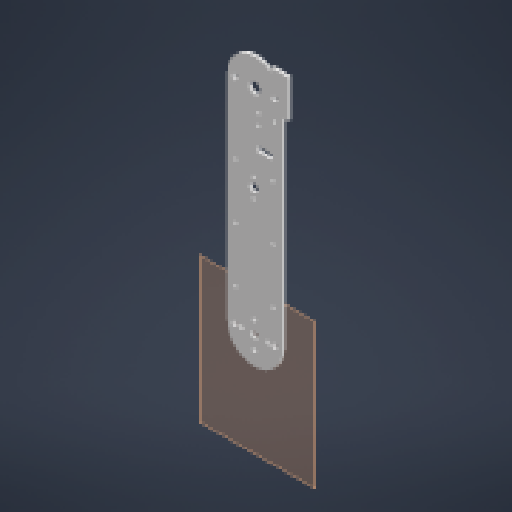
# Autodesk Inventor part: Link2Base
Saved by Autodesk Inventor 2023 (Build 270158000, 158)
## iProperties
Created: 2023-09-09
Part Number: Link2Base
Material: Generic
Document SubType Name: Modeling
Designer: philo
Density: 1 g/cm^3
Appearance: Default
Author: philo
Autodesk Inventor part; units mm, degrees
ref_plane "YZ Plane" through (0, 0, 0) normal (1, 0, 0) x (0, 1, 0)
ref_plane "XZ Plane" through (0, 0, 0) normal (0, 1, 0) x (-1, 0, 0)
ref_plane "XY Plane" through (0, 0, 0) normal (0, 0, 1) x (1, 0, 0)
ref_plane "Work Plane2" through (0.4904, 0, 14) normal (0, 0, 1) x (1, 0, 0)
sketch "Sketch1" plane through (0.4904, 0, 14) normal (0, 0, 1) x (1, 0, 0)
  line L0 (-25, 225.7065) -> (25, 225.7065)
  line L1 (25, 225.7065) -> (25, 5.7065)
  line L2 (25, 5.7065) -> (-25, 5.7065)
  line L3 (-25, 5.7065) -> (-25, 225.7065)
  line L4 (-25, 225.7065) -> (25, 225.7065)
  line L5 (20, 5.7065) -> (-20, 5.7065)
  circle A0 centre (0, 30.7065) radius 3.5 projected
  circle A1 centre (0, 30.7065) radius 25
  circle A2 centre (0, 225.7065) radius 25
  line L6 (-25, 30.7065) -> (-25, 225.7065)
  line L7 (25, 225.7065) -> (25, 30.7065)
  point P0 (-0.4904, 0)
  dimension "d19" = 50
  dimension "d6" = 220
  dimension "d7" = 0
  dimension "d9" = 50
  dimension "d10" = 25
  dimension "d11" = 25
  dimension "d12" = 25
  dimension "d13" = 0
  constraints: 16 end point, 3 parallel, 2 horizontal, 2 point on circle, 2 point on line, 1 centre point, 1 coincident, 1 midpoint, 1 perpendicular, 3 other
  measures "d6" distance between parallel lines of L2 L0
  measures "d7" distance between parallel lines of L0 L4
  measures "d9" diameter of A1
  measures "d10" distance from line of L3 A1.centre
  measures "d11" distance from line of L1 A1.centre
  measures "d12" distance from line of A1.centre L2
  measures "d13" distance between parallel lines of L5 L2
extrude "Extrusion1" add sketch "Sketch1" along normal blind 3 contours A2 L0 | A2 L1 A1 L3 | L0 A2 | A1
sketch "Sketch2" plane through (0.4904, 0, 17) normal (0, 0, 1) x (1, 0, 0)
  arc A0 (25, 225.7065) -> (-25, 225.7065) centre (0, 225.7065) ccw projected
  circle A1 centre (0, 225.7065) radius 5
  point P0 (-0.4904, 0)
  dimension "d16" = 10
  constraints: 1 centre point, 1 coincident
  measures "d16" diameter of A1
extrude "Extrusion2" cut sketch "Sketch2" against normal blind 3
sketch "Sketch4" plane through (0.4904, 0, 17) normal (0, 0, 1) x (1, 0, 0)
  arc A0 (20.4946, 25.2317) -> (20.5054, 36.1404) centre (18, 30.6886) ccw projected
  line L0 (20.5054, 36.1404) -> (10.4453, 40.7636) projected
  arc A1 (10.4252, 20.6286) -> (10.4453, 40.7636) centre (0, 30.7065) ccw projected
  line L1 (10.4252, 20.6286) -> (20.4946, 25.2317) projected
  circle A2 centre (18, 30.6886) radius 2.5 projected
  arc A3 (-20.5376, 36.019) -> (-20.4622, 25.1105) centre (-18, 30.582) ccw projected
  line L2 (-20.4622, 25.1105) -> (-11.0226, 20.8627) projected
  arc A4 (-11.1577, 40.3969) -> (-11.0226, 20.8627) centre (0, 30.7065) ccw projected
  line L3 (-11.1577, 40.3969) -> (-20.5376, 36.019) projected
  circle A5 centre (-18, 30.582) radius 2.5 projected
  point P0 (-0.4904, 0)
extrude "Extrusion4" cut sketch "Sketch4" against normal blind 10 contours A2 | A5
sketch "Sketch6" plane through (0.4904, 0, 14) normal (0, 0, -1) x (-1, 0, 0)
  circle A0 centre (0, 42.7065) radius 2 projected
  circle A1 centre (-12, 30.7065) radius 2 projected
  circle A2 centre (0, 18.7065) radius 2 projected
  circle A3 centre (12, 30.7065) radius 2 projected
  point P0 (0.4904, 0)
extrude "Extrusion6" cut sketch "Sketch6" against normal blind 10
sketch "Sketch7" plane through (0.4904, 0, 14) normal (0, 0, -1) x (-1, 0, 0)
  circle A0 centre (-12, 30.7065) radius 2 projected
  circle A1 centre (0, 18.7065) radius 2 projected
  circle A2 centre (12, 30.7065) radius 2 projected
  circle A3 centre (0, 42.7065) radius 2 projected
  circle A4 centre (-18, 30.6886) radius 2.5 projected
  circle A5 centre (18, 30.582) radius 2.5 projected
  circle A6 centre (0, 225.7065) radius 5 projected
  line L0 (25, 225.7065) -> (25, 30.7065) projected
  line L1 (-25, 30.7065) -> (-25, 225.7065) projected
  arc A7 (-25, 30.7065) -> (25, 30.7065) centre (0, 30.7065) ccw projected
  circle A8 centre (0, 30.7065) radius 3.5 projected
  circle A9 centre (0.668, 146.5279) radius 12.5 projected
  circle A10 centre (9.168, 146.5279) radius 2.3813 projected
  circle A11 centre (-7.832, 146.5279) radius 2.3813 projected
  circle A12 centre (0.668, 155.0279) radius 1.5 projected
  circle A13 centre (0.668, 138.0279) radius 1.5 projected
  circle A14 centre (0.668, 146.5279) radius 4
  arc A15 (25, 225.7065) -> (-25, 225.7065) centre (0, 225.7065) ccw projected
  point P0 (0.4904, 0)
  dimension "d60" = 8
  constraints: 1 centre point, 1 coincident
  measures "d60" diameter of A14
extrude "Extrusion7" cut sketch "Sketch7" against normal blind 10 contours A12 | A13 | A14
sketch "Sketch10" plane through (0.4904, 0, 17) normal (0, 0, 1) x (1, 0, 0)
  line L0 (17, 181.6543) -> (2, 181.6543)
  line L1 (2, 181.6543) -> (2, 176.6543)
  line L2 (2, 176.6543) -> (17, 176.6543)
  line L3 (17, 176.6543) -> (17, 181.6543)
  line L4 (25, 30.7065) -> (25, 225.7065) projected
  point P0 (-0.4904, 0)
  dimension "d67" = 15
  dimension "d68" = 5
  dimension "d69" = 8
  constraints: 8 end point, 2 parallel, 1 horizontal, 1 perpendicular
  measures "d67" distance of L2.end L1.end
  measures "d68" distance of L1.end L0.end
  measures "d69" distance between parallel lines of L4 L3
extrude "Extrusion10" cut sketch "Sketch10" against normal blind 10
fillet "Fillet1" radius 2 4 edges at (17.4904, 176.6543, 15.5) (17.4904, 181.6543, 15.5) (2.4904, 181.6543, 15.5) (2.4904, 176.6543, 15.5)
sketch "Sketch11" plane through (0.4904, 0, 17) normal (0, 0, 1) x (1, 0, 0)
  arc A0 (20.5376, 220.3941) -> (20.4622, 231.3026) centre (18, 225.831) ccw projected
  line L0 (20.4622, 231.3026) -> (11.0226, 235.5503) projected
  arc A1 (11.1577, 216.0162) -> (11.0226, 235.5503) centre (0, 225.7065) ccw projected
  line L1 (11.1577, 216.0162) -> (20.5376, 220.3941) projected
  circle A2 centre (18, 225.831) radius 2.5 projected
  arc A3 (-20.4946, 231.1813) -> (-20.5054, 220.2726) centre (-18, 225.7245) ccw projected
  line L2 (-20.5054, 220.2726) -> (-10.4453, 215.6494) projected
  arc A4 (-10.4252, 235.7844) -> (-10.4453, 215.6494) centre (0, 225.7065) ccw projected
  line L3 (-10.4252, 235.7844) -> (-20.4946, 231.1813) projected
  circle A5 centre (-18, 225.7245) radius 2.5 projected
  circle A6 centre (3.5, 208.0565) radius 1.5 projected
  circle A7 centre (3.5, 197.2565) radius 1.5 projected
  line L4 (15, 176.6543) -> (4, 176.6543) projected
  arc A8 (2, 178.6543) -> (4, 176.6543) centre (4, 178.6543) ccw projected
  line L5 (2, 178.6543) -> (2, 179.6543) projected
  arc A9 (4, 181.6543) -> (2, 179.6543) centre (4, 179.6543) ccw projected
  line L6 (4, 181.6543) -> (15, 181.6543) projected
  arc A10 (17, 179.6543) -> (15, 181.6543) centre (15, 179.6543) ccw projected
  line L7 (17, 179.6543) -> (17, 178.6543) projected
  arc A11 (15, 176.6543) -> (17, 178.6543) centre (15, 178.6543) ccw projected
  circle A12 centre (-0.668, 146.5279) radius 4 projected
  circle A13 centre (-0.668, 138.0279) radius 1.5 projected
  circle A14 centre (-0.668, 155.0279) radius 1.5 projected
  circle A15 centre (12, 30.7065) radius 2 projected
  circle A16 centre (0, 18.7065) radius 2 projected
  circle A17 centre (-12, 30.7065) radius 2 projected
  circle A18 centre (0, 42.7065) radius 2 projected
  circle A19 centre (18, 30.6886) radius 2.5 projected
  circle A20 centre (-18, 30.582) radius 2.5 projected
  circle A21 centre (0, 225.7065) radius 5 projected
  line L8 (-25, 225.7065) -> (-25, 30.7065) projected
  arc A22 (-25, 30.7065) -> (25, 30.7065) centre (0, 30.7065) ccw projected
  line L9 (25, 30.7065) -> (25, 225.7065) projected
  arc A23 (25, 225.7065) -> (-25, 225.7065) centre (0, 225.7065) ccw projected
  circle A24 centre (0, 30.7065) radius 3.5 projected
  circle A25 centre (18.3, 208.0565) radius 1.5 projected
  point P0 (-0.4904, 0)
extrude "Extrusion11" cut sketch "Sketch11" against normal blind 10 contours A2 | A5
sketch "Sketch12" plane through (0.4904, 0, 17) normal (0, 0, 1) x (1, 0, 0)
  circle A0 centre (17, 60.7065) radius 1.5
  circle A1 centre (-17, 60.7065) radius 1.5
  circle A2 centre (-17, 110.7065) radius 1.5
  circle A3 centre (17, 110.7065) radius 1.5
  circle A4 centre (-17, 160.7065) radius 1.5
  line L0 (-25, 225.7065) -> (-25, 30.7065) projected
  line L1 (25, 30.7065) -> (25, 225.7065) projected
  circle A5 centre (0, 30.7065) radius 3.5 projected
  circle A6 centre (17, 160.7065) radius 1.5
  point P0 (-0.4904, 0)
  dimension "d75" = 3
  dimension "d76" = 3
  dimension "d77" = 3
  dimension "d78" = 3
  dimension "d79" = 3
  dimension "d80" = 8
  dimension "d81" = 8
  dimension "d82" = 8
  dimension "d83" = 8
  dimension "d84" = 8
  dimension "d85" = 30
  dimension "d86" = 30
  dimension "d87" = 50
  dimension "d88" = 50
  dimension "d89" = 50
  dimension "d90" = 3
  dimension "d91" = 8
  dimension "d92" = 50
  constraints: 6 centre point
  measures "d75" diameter of A0
  measures "d76" diameter of A1
  measures "d77" diameter of A2
  measures "d78" diameter of A3
  measures "d79" diameter of A4
  measures "d80" distance from line of L0 A1.centre
  measures "d81" distance from line of L1 A0.centre
  measures "d82" distance from line of L1 A3.centre
  measures "d83" distance from line of L0 A2.centre
  measures "d84" distance from line of L0 A4.centre
  measures "d85" vertical distance of A5.centre A0.centre
  measures "d86" vertical distance of A5.centre A1.centre
  measures "d87" distance of A3.centre A0.centre
  measures "d88" distance of A2.centre A1.centre
  measures "d89" distance of A4.centre A2.centre
  measures "d90" diameter of A6
  measures "d91" distance from line of L1 A6.centre
  measures "d92" distance of A3.centre A6.centre
extrude "Extrusion12" cut sketch "Sketch12" against normal blind 10 contours A0 | A1 | A2 | A3 | A4 | A6
sketch "Sketch13" plane through (0.4904, 0, 17) normal (0, 0, 1) x (1, 0, 0)
  line L0 (15.5, 214.3827) -> (30.5, 214.3827)
  line L1 (30.5, 214.3827) -> (30.5, 249.3827)
  line L2 (30.5, 249.3827) -> (15.5, 249.3827)
  line L3 (15.5, 249.3827) -> (15.5, 214.3827)
  circle A0 centre (18, 225.831) radius 2.5 projected
  point P0 (-0.4904, 0)
  point P1 (15.5, 225.831)
  dimension "d95" = 15
  dimension "d96" = 35
  constraints: 8 end point, 2 parallel, 1 horizontal, 1 perpendicular
  measures "d95" distance of L2.end L1.end
  measures "d96" distance of L1.end L0.end
extrude "Extrusion13" add sketch "Sketch13" against normal blind 3
sketch "Sketch14" plane through (0.4904, 0, 14) normal (0, 0, -1) x (-1, 0, 0)
  circle A0 centre (-18.15, 246.2827) radius 1.5 projected
  circle A1 centre (-18.15, 212.3827) radius 1.5 projected
  circle A2 centre (-28.95, 212.3827) radius 1.5 projected
  point P0 (0.4904, 0)
extrude "Extrusion14" cut sketch "Sketch14" against normal blind 3 contours A0 | A1
fillet "Fillet2" radius 3 5 edges at (15.9904, 245.3216, 15.5) (15.9904, 249.3827, 15.5) (30.9904, 249.3827, 15.5) (30.9904, 214.3827, 15.5) (25.4904, 214.3827, 15.5)
body "Solid1"
